Autodesk Fusion 360 part; units mm, degrees
(part 4 of 13)
  line L2684 (147.36, -101.854) -> (147.266, -101.874)
  line L2685 (145.516, -107.036) -> (145.448, -107.016)
  line L2686 (147.651, -101.836) -> (147.644, -101.834)
  line L2687 (148.011, -101.956) -> (148.011, -101.956)
  line L2688 (147.957, -106.91) -> (147.936, -106.978)
  line L2689 (147.447, -101.836) -> (147.36, -101.854)
  line L2690 (147.644, -101.834) -> (147.453, -101.834)
  line L2691 (147.999, -101.949) -> (147.999, -101.949)
  line L2692 (147.098, -101.949) -> (147.098, -101.949)
  line L2693 (147.651, -101.836) -> (147.651, -101.836)
  line L2694 (146.733, -102.004) -> (146.733, -102.004)
  line L2695 (146.733, -102.004) -> (146.727, -102.001)
  line L2696 (148.005, -101.952) -> (147.999, -101.949)
  line L2697 (146.727, -102.001) -> (146.633, -101.981)
  line L2698 (147.453, -101.834) -> (147.447, -101.836)
  line L2699 (146.342, -103.777) -> (146.349, -103.778)
  line L2700 (146.405, -103.778) -> (146.473, -103.799)
  line L2701 (146.349, -103.778) -> (146.405, -103.778)
  line L2702 (146.546, -101.963) -> (146.546, -101.963)
  line L2703 (147.936, -106.978) -> (147.883, -107.024)
  line L2704 (146.342, -101.963) -> (146.342, -101.963)
  line L2705 (145.448, -107.016) -> (145.402, -106.962)
  line L2706 (145.402, -106.962) -> (145.392, -106.892)
  line L2707 (146.255, -103.759) -> (146.342, -103.777)
  line L2708 (146.156, -103.736) -> (146.162, -103.739)
  line L2709 (145.844, -103.557) -> (145.988, -103.661)
  line L2710 (146.224, -101.988) -> (145.844, -102.369)
  line L2711 (146.54, -101.962) -> (146.349, -101.962)
  line L2712 (145.844, -102.369) -> (145.844, -103.557)
  line L2713 (146.473, -103.799) -> (146.494, -103.815)
  line L2714 (146.255, -101.981) -> (146.224, -101.988)
  line L2715 (146.546, -101.963) -> (146.54, -101.962)
  line L2716 (145.994, -103.664) -> (146.156, -103.736)
  line L2717 (146.342, -101.963) -> (146.255, -101.981)
  line L2718 (146.162, -103.739) -> (146.255, -103.759)
  line L2719 (146.342, -103.777) -> (146.342, -103.777)
  line L2720 (145.419, -106.809) -> (145.425, -106.765)
  line L2721 (146.173, -98.3593) -> (146.176, -98.3565)
  line L2722 (145.404, -106.846) -> (145.411, -106.828)
  line L2723 (145.994, -103.664) -> (145.994, -103.664)
  line L2724 (145.401, -106.858) -> (145.404, -106.846)
  line L2725 (145.415, -106.816) -> (145.419, -106.809)
  line L2726 (145.425, -106.765) -> (145.428, -106.754)
  line L2727 (145.398, -106.868) -> (145.399, -106.866)
  line L2728 (150.849, -79.1963) -> (150.82, -79.1551)
  line L2729 (150.946, -80.2588) -> (151.001, -80.0568)
  line L2730 (150.485, -80.0187) -> (150.435, -80.1497)
  line L2731 (150.946, -79.4056) -> (150.943, -79.3953)
  line L2732 (151.021, -79.8267) -> (151.002, -79.6184)
  line L2733 (150.821, -80.5085) -> (150.849, -80.4681)
  line L2734 (150.81, -79.1467) -> (150.796, -79.1537)
  line L2735 (151.002, -79.6184) -> (151.001, -79.6076)
  line L2736 (144.637, -93.3612) -> (144.728, -93.5556)
  line L2737 (144.879, -93.7872) -> (144.882, -93.7913)
  line L2738 (151.001, -79.6076) -> (150.946, -79.4056)
  line L2739 (144.568, -93.1202) -> (144.607, -93.2578)
  line L2740 (148.43, -96.7994) -> (148.43, -96.8204)
  line L2741 (148.43, -96.8204) -> (148.415, -96.8969)
  line L2742 (144.635, -93.3566) -> (144.637, -93.3612)
  line L2743 (144.607, -93.2578) -> (144.635, -93.3566)
  line L2744 (148.284, -97.5103) -> (148.289, -97.5255)
  line L2745 (144.637, -93.3612) -> (144.637, -93.3612)
  line L2746 (144.728, -93.5556) -> (144.741, -93.5839)
  line L2747 (144.744, -93.5881) -> (144.744, -93.5881)
  line L2748 (150.854, -80.4586) -> (150.943, -80.2691)
  line L2749 (150.797, -80.5114) -> (150.809, -80.5178)
  line L2750 (144.741, -93.5839) -> (144.744, -93.5881)
  line L2751 (145.25, -94.1228) -> (145.25, -94.1228)
  line L2752 (144.744, -93.5881) -> (144.879, -93.7872)
  line L2753 (150.796, -79.1537) -> (150.437, -79.5133)
  line L2754 (151.002, -80.046) -> (151.021, -79.8377)
  line L2755 (150.437, -79.5133) -> (150.49, -79.666)
  line L2756 (150.508, -79.8531) -> (150.485, -80.0187)
  line L2757 (150.809, -80.5178) -> (150.821, -80.5085)
  line L2758 (151.001, -80.0568) -> (151.002, -80.046)
  line L2759 (144.568, -93.1202) -> (144.568, -93.1202)
  line L2760 (146.166, -94.3699) -> (146.166, -94.3699)
  line L2761 (145.815, -94.3439) -> (145.955, -94.3681)
  line L2762 (146.346, -94.3555) -> (146.346, -94.3555)
  line L2763 (146.346, -94.3555) -> (146.351, -94.3551)
  line L2764 (145.988, -94.37) -> (145.988, -94.37)
  line L2765 (145.475, -94.2444) -> (145.48, -94.246)
  line L2766 (146.351, -94.3551) -> (146.356, -94.3539)
  line L2767 (150.943, -80.2691) -> (150.946, -80.2588)
  line L2768 (150.435, -80.1497) -> (150.797, -80.5114)
  line L2769 (150.943, -79.3953) -> (150.854, -79.2058)
  line L2770 (146.166, -94.3699) -> (146.346, -94.3555)
  line L2771 (145.329, -94.1662) -> (145.475, -94.2444)
  line L2772 (150.854, -79.2058) -> (150.849, -79.1963)
  line L2773 (144.882, -93.7913) -> (144.886, -93.795)
  line L2774 (145.712, -94.326) -> (145.815, -94.3439)
  line L2775 (151.021, -79.8377) -> (151.021, -79.8267)
  line L2776 (150.82, -79.1551) -> (150.81, -79.1467)
  line L2777 (150.849, -80.4681) -> (150.854, -80.4586)
  line L2778 (148.307, -97.0052) -> (148.284, -97.0097)
  line L2779 (144.879, -93.7872) -> (144.879, -93.7872)
  circle A28 centre (112.573, -110.134) radius 0.2
  circle A29 centre (123.749, -107.996) radius 0.2
  circle A30 centre (148.895, -97.028) radius 0.2
  circle A31 centre (115.214, -116.18) radius 0.2
  circle A32 centre (123.774, -112.954) radius 0.2
  circle A33 centre (92.8116, -81.2546) radius 0.2
  circle A34 centre (110.388, -108.255) radius 0.2
  circle A35 centre (131.47, -114.3) radius 0.2
  circle A36 centre (130.531, -107.975) radius 0.2
  circle A37 centre (137.897, -112.624) radius 0.2
  circle A38 centre (133.429, -109.717) radius 0.2
  circle A39 centre (150.622, -97.3582) radius 0.2
  circle A40 centre (128.067, -87.2236) radius 0.2
  circle A41 centre (146.228, -106.299) radius 0.2
  circle A42 centre (127.254, -107.061) radius 0.2
  circle A43 centre (115.113, -71.9328) radius 0.2
  circle A44 centre (105.74, -104.191) radius 0.2
  circle A45 centre (92.4814, -111.887) radius 0.2
  circle A46 centre (122.123, -94.5134) radius 0.2
  circle A47 centre (141.061, -112.152) radius 0.2
  circle A48 centre (92.4306, -104.216) radius 0.2
  circle A49 centre (115.214, -113.411) radius 0.2
  circle A50 centre (126.187, -110.49) radius 0.2
  circle A51 centre (126.749, -94.435) radius 0.2
  circle A52 centre (117.291, -131.755) radius 0.2
  circle A53 centre (136.169, -97.9424) radius 0.2
  circle A54 centre (138.735, -98.0186) radius 0.2
  circle A55 centre (132.232, -94.8763) radius 0.2
  circle A56 centre (147.701, -101.067) radius 0.2
  circle A57 centre (149.463, -102.253) radius 0.2
  circle A58 centre (144.958, -107.874) radius 0.2
  circle A59 centre (149.925, -95.573) radius 0.2
  circle A60 centre (123.901, -94.5134) radius 0.2
  circle A61 centre (147.549, -102.743) radius 0.2
  line L2780 (104.259, -121.194) -> (104.353, -121.345)
  circle A62 centre (126.543, -112.471) radius 0.2
  line L2781 (104.133, -121.067) -> (104.259, -121.194)
  line L2782 (104.132, -121.066) -> (104.133, -121.067)
  line L2783 (106.931, -109.689) -> (106.934, -109.709)
  line L2784 (106.805, -115.238) -> (104.132, -117.911)
  line L2785 (106.805, -109.476) -> (106.809, -109.48)
  line L2786 (106.809, -109.48) -> (106.839, -109.522)
  line L2787 (106.873, -109.56) -> (106.881, -109.579)
  line L2788 (106.951, -109.83) -> (106.951, -114.884)
  line L2789 (106.934, -109.709) -> (106.941, -109.728)
  line L2790 (106.951, -114.89) -> (106.944, -114.941)
  line L2791 (105.52, -108.191) -> (106.805, -109.476)
  line L2792 (106.869, -115.159) -> (106.836, -115.197)
  line L2793 (104.132, -117.911) -> (104.132, -121.066)
  line L2794 (106.951, -114.884) -> (106.951, -114.89)
  line L2795 (106.93, -115.03) -> (106.908, -115.077)
  line L2796 (106.881, -109.579) -> (106.893, -109.595)
  line L2797 (106.878, -115.14) -> (106.869, -115.159)
  line L2798 (106.94, -114.992) -> (106.933, -115.01)
  line L2799 (106.933, -115.01) -> (106.93, -115.03)
  line L2800 (106.941, -109.728) -> (106.944, -109.779)
  line L2801 (106.944, -114.941) -> (106.94, -114.992)
  line L2802 (103.077, -107.563) -> (103.096, -107.57)
  line L2803 (105.293, -108.064) -> (105.313, -108.067)
  line L2804 (107.04, -125.464) -> (107.072, -125.472)
  line L2805 (143.674, -125.474) -> (143.701, -125.474)
  line L2806 (106.992, -125.455) -> (106.992, -125.455)
  line L2807 (103.244, -107.634) -> (103.282, -107.667)
  line L2808 (105.441, -108.127) -> (105.479, -108.161)
  line L2809 (106.89, -115.124) -> (106.878, -115.14)
  line L2810 (106.893, -109.595) -> (106.91, -109.643)
  line L2811 (103.026, -107.559) -> (103.077, -107.563)
  line L2812 (143.609, -125.476) -> (143.609, -125.476)
  line L2813 (104.245, -122.205) -> (104.132, -122.312)
  line L2814 (143.583, -125.474) -> (143.594, -125.475)
  line L2815 (143.594, -125.475) -> (143.602, -125.477)
  line L2816 (106.944, -109.779) -> (106.951, -109.83)
  line L2817 (103.608, -107.982) -> (104.088, -107.982)
  line L2818 (105.223, -108.053) -> (105.274, -108.057)
  line L2819 (104.088, -107.982) -> (104.184, -108.001)
  line L2820 (107.072, -125.472) -> (107.083, -125.474)
  line L2821 (106.984, -125.454) -> (106.992, -125.455)
  line L2822 (106.992, -125.455) -> (107.028, -125.461)
  line L2823 (106.91, -109.643) -> (106.931, -109.689)
  line L2824 (104.132, -122.615) -> (106.962, -125.445)
  line L2825 (106.908, -115.077) -> (106.89, -115.124)
  line L2826 (103.116, -107.573) -> (103.162, -107.595)
  line L2827 (107.169, -125.477) -> (107.187, -125.475)
  line L2828 (103.21, -107.613) -> (103.226, -107.625)
  line L2829 (103.226, -107.625) -> (103.244, -107.634)
  line L2830 (104.353, -121.345) -> (104.412, -121.513)
  line L2831 (96.4732, -107.552) -> (96.4732, -107.502)
  line L2832 (107.198, -125.474) -> (143.583, -125.474)
  line L2833 (105.359, -108.088) -> (105.407, -108.106)
  line L2834 (104.184, -108.001) -> (104.249, -108.045)
  line L2835 (105.274, -108.057) -> (105.293, -108.064)
  line L2836 (105.167, -108.045) -> (105.173, -108.045)
  line L2837 (105.479, -108.161) -> (105.52, -108.191)
  line L2838 (104.249, -108.045) -> (105.167, -108.045)
  line L2839 (107.103, -125.474) -> (107.123, -125.476)
  line L2840 (104.407, -121.89) -> (104.344, -122.056)
  line L2841 (107.187, -125.475) -> (107.198, -125.474)
  line L2842 (103.162, -107.595) -> (103.21, -107.613)
  line L2843 (104.412, -121.513) -> (104.432, -121.691)
  line L2844 (105.313, -108.067) -> (105.359, -108.088)
  line L2845 (101.073, -107.552) -> (102.97, -107.552)
  line L2846 (105.173, -108.045) -> (105.223, -108.053)
  line L2847 (106.839, -109.522) -> (106.873, -109.56)
  line L2848 (107.15, -125.478) -> (107.169, -125.477)
  line L2849 (143.602, -125.477) -> (143.609, -125.476)
  line L2850 (103.282, -107.667) -> (103.323, -107.698)
  line L2851 (143.67, -125.475) -> (143.674, -125.474)
  line L2852 (94.3232, -107.552) -> (96.4732, -107.552)
  line L2853 (107.083, -125.474) -> (107.103, -125.474)
  line L2854 (103.096, -107.57) -> (103.116, -107.573)
  line L2855 (106.836, -115.197) -> (106.805, -115.238)
  line L2856 (107.143, -125.479) -> (107.15, -125.478)
  line L2857 (107.028, -125.461) -> (107.04, -125.464)
  line L2858 (102.976, -107.552) -> (103.026, -107.559)
  line L2859 (105.423, -108.118) -> (105.441, -108.127)
  line L2860 (143.609, -125.476) -> (143.67, -125.475)
  line L2861 (103.323, -107.698) -> (103.608, -107.982)
  line L2862 (101.073, -107.502) -> (101.073, -107.552)
  line L2863 (96.4732, -107.502) -> (101.073, -107.502)
  line L2864 (102.97, -107.552) -> (102.976, -107.552)
  line L2865 (105.407, -108.106) -> (105.423, -108.118)
  line L2866 (104.432, -121.713) -> (104.407, -121.89)
  line L2867 (147.946, -122.352) -> (147.95, -122.347)
  line L2868 (144.084, -125.317) -> (144.099, -125.306)
  line L2869 (147.652, -122.7) -> (147.656, -122.697)
  line L2870 (146.52, -122.967) -> (146.579, -122.983)
  line L2871 (143.8, -125.462) -> (143.813, -125.46)
  line L2872 (143.969, -125.401) -> (143.99, -125.386)
  line L2873 (147.83, -122.518) -> (147.946, -122.352)
  line L2874 (143.75, -125.472) -> (143.754, -125.472)
  line L2875 (147.464, -122.83) -> (147.469, -122.828)
  line L2876 (143.922, -125.423) -> (143.933, -125.417)
  line L2877 (147.261, -122.925) -> (147.304, -122.905)
  line L2878 (143.754, -125.472) -> (143.761, -125.472)
  line L2879 (147.952, -122.342) -> (147.952, -122.342)
  line L2880 (147.818, -122.535) -> (147.83, -122.518)
  line L2881 (143.873, -125.439) -> (143.908, -125.429)
  line L2882 (106.962, -125.445) -> (106.966, -125.446)
  line L2883 (143.761, -125.472) -> (143.781, -125.466)
  line L2884 (144.082, -125.318) -> (144.084, -125.317)
  line L2885 (144.015, -125.368) -> (144.046, -125.35)
  line L2886 (147.656, -122.697) -> (147.818, -122.535)
  line L2887 (146.579, -122.983) -> (146.584, -122.984)
  line L2888 (147.594, -122.741) -> (147.652, -122.7)
  line L2889 (143.781, -125.466) -> (143.8, -125.462)
  line L2890 (143.828, -125.457) -> (143.862, -125.443)
  line L2891 (146.584, -122.984) -> (146.812, -123.004)
  line L2892 (143.99, -125.386) -> (144.005, -125.375)
  line L2893 (143.705, -125.474) -> (143.705, -125.474)
  line L2894 (147.304, -122.905) -> (147.464, -122.83)
  line L2895 (143.908, -125.429) -> (143.908, -125.429)
  line L2896 (143.915, -125.427) -> (143.922, -125.423)
  line L2897 (104.132, -122.312) -> (104.132, -122.615)
  line L2898 (104.344, -122.056) -> (104.245, -122.205)
  line L2899 (147.952, -122.342) -> (148.044, -122.145)
  line L2900 (107.123, -125.476) -> (107.143, -125.479)
  line L2901 (143.828, -125.457) -> (143.828, -125.457)
  line L2902 (143.95, -125.408) -> (143.969, -125.401)
  line L2903 (146.812, -123.004) -> (147.04, -122.984)
  line L2904 (143.705, -125.474) -> (143.717, -125.473)
  line L2905 (144.046, -125.35) -> (144.053, -125.346)
  line L2906 (148.044, -122.145) -> (148.044, -122.145)
  line L2907 (147.04, -122.984) -> (147.045, -122.983)
  line L2908 (104.432, -121.691) -> (104.432, -121.713)
  line L2909 (144.053, -125.346) -> (144.067, -125.331)
  line L2910 (106.966, -125.446) -> (106.984, -125.454)
  line L2911 (143.813, -125.46) -> (143.813, -125.46)
  line L2912 (147.045, -122.983) -> (147.256, -122.926)
  line L2913 (143.933, -125.417) -> (143.95, -125.408)
  line L2914 (143.82, -125.459) -> (143.828, -125.457)
  line L2915 (144.067, -125.331) -> (144.082, -125.318)
  line L2916 (144.127, -125.272) -> (144.135, -125.264)
  line L2917 (147.652, -122.7) -> (147.652, -122.7)
  line L2918 (144.046, -125.35) -> (144.046, -125.35)
  line L2919 (143.862, -125.443) -> (143.873, -125.439)
  line L2920 (143.717, -125.473) -> (143.75, -125.472)
  line L2921 (146.399, -123) -> (146.461, -122.966)
  line L2922 (147.256, -122.926) -> (147.261, -122.925)
  line L2923 (143.908, -125.429) -> (143.915, -125.427)
  line L2924 (143.701, -125.474) -> (143.705, -125.474)
  line L2925 (143.922, -125.423) -> (143.922, -125.423)
  line L2926 (144.005, -125.375) -> (144.015, -125.368)
  line L2927 (143.813, -125.46) -> (143.82, -125.459)
  line L2928 (144.099, -125.306) -> (144.127, -125.272)
  line L2929 (144.135, -125.264) -> (146.399, -123)
  line L2930 (150.834, -138.766) -> (150.829, -138.766)
  line L2931 (151.926, -138.995) -> (151.705, -138.877)
  line L2932 (151.191, -138.751) -> (151.016, -138.751)
  line L2933 (150.67, -138.805) -> (150.586, -138.826)
  line L2934 (151.7, -138.875) -> (151.473, -138.797)
  line L2935 (147.95, -121.034) -> (147.837, -120.874)
  line L2936 (151.365, -138.777) -> (151.225, -138.753)
  line L2937 (151.93, -138.998) -> (151.93, -138.998)
  line L2938 (152.509, -139.452) -> (152.439, -139.463)
  line L2939 (152.562, -139.405) -> (152.509, -139.452)
  line L2940 (147.884, -120.689) -> (147.941, -120.675)
  line L2941 (147.952, -121.039) -> (147.95, -121.034)
  line L2942 (146.461, -122.966) -> (146.52, -122.967)
  line L2943 (152.351, -139.409) -> (152.301, -139.334)
  line L2944 (152.439, -139.463) -> (152.374, -139.434)
  line L2945 (148.106, -121.919) -> (148.125, -121.691)
  line L2946 (147.469, -122.828) -> (147.594, -122.741)
  line L2947 (147.952, -121.039) -> (147.952, -121.039)
  line L2948 (147.832, -120.738) -> (147.884, -120.689)
  line L2949 (148.125, -121.691) -> (148.106, -121.463)
  line L2950 (152.301, -139.334) -> (152.298, -139.33)
  line L2951 (150.581, -138.828) -> (150.581, -138.828)
  line L2952 (151.221, -138.752) -> (151.217, -138.752)
  line L2953 (152.298, -139.33) -> (152.197, -139.223)
  line L2954 (152.455, -124.205) -> (152.582, -139.337)
  line L2955 (151.473, -138.797) -> (151.468, -138.795)
  line L2956 (147.815, -120.806) -> (147.832, -120.738)
  line L2957 (152.197, -139.223) -> (152.129, -139.151)
  line L2958 (151.7, -138.875) -> (151.7, -138.875)
  line L2959 (148.044, -122.145) -> (148.046, -122.14)
  line L2960 (152.426, -120.8) -> (152.455, -124.205)
  line L2961 (151.225, -138.753) -> (151.221, -138.752)
  line L2962 (151.468, -138.795) -> (151.365, -138.777)
  line L2963 (150.834, -138.766) -> (150.834, -138.766)
  line L2964 (147.045, -122.983) -> (147.045, -122.983)
  line L2965 (147.95, -122.347) -> (147.952, -122.342)
  line L2966 (152.374, -139.434) -> (152.351, -139.409)
  line L2967 (150.581, -138.828) -> (150.46, -138.879)
  line L2968 (152.369, -120.695) -> (152.415, -120.749)
  line L2969 (152.071, -139.106) -> (151.93, -138.998)
  line L2970 (151.217, -138.752) -> (151.217, -138.752)
  line L2971 (147.256, -122.926) -> (147.256, -122.926)
  line L2972 (148.046, -121.241) -> (147.968, -121.073)
  line L2973 (147.941, -120.675) -> (152.3, -120.675)
  line L2974 (150.824, -138.767) -> (150.67, -138.805)
  line L2975 (150.586, -138.826) -> (150.581, -138.828)
  line L2976 (146.579, -122.983) -> (146.579, -122.983)
  line L2977 (147.968, -121.073) -> (147.952, -121.039)
  line L2978 (152.3, -120.675) -> (152.369, -120.695)
  line L2979 (152.415, -120.749) -> (152.426, -120.8)
  line L2980 (151.016, -138.751) -> (151.014, -138.751)
  line L2981 (148.106, -121.463) -> (148.046, -121.241)
  line L2982 (152.582, -139.337) -> (152.562, -139.405)
  line L2983 (148.046, -122.14) -> (148.106, -121.919)
  line L2984 (151.192, -138.751) -> (151.191, -138.751)
  line L2985 (150.829, -138.766) -> (150.824, -138.767)
  line L2986 (152.129, -139.151) -> (152.125, -139.148)
  line L2987 (152.125, -139.148) -> (152.071, -139.106)
  line L2988 (151.014, -138.751) -> (151.014, -138.751)
  line L2989 (147.837, -120.874) -> (147.815, -120.806)
  line L2990 (147.464, -122.83) -> (147.464, -122.83)
  line L2991 (151.705, -138.877) -> (151.7, -138.875)
  line L2992 (151.014, -138.751) -> (150.834, -138.766)
  line L2993 (149.864, -141.293) -> (149.964, -141.399)
  line L2994 (150.369, -141.781) -> (150.345, -141.848)
  line L2995 (149.616, -140.859) -> (149.616, -140.859)
  line L2996 (149.528, -140.114) -> (149.528, -140.119)
  line L2997 (97.264, -141.636) -> (97.2177, -141.582)
  line L2998 (150.037, -141.475) -> (150.037, -141.475)
  line L2999 (97.2131, -140.453) -> (97.2139, -140.314)
  line L3000 (150.037, -141.475) -> (150.228, -141.621)
  line L3001 (151.93, -138.998) -> (151.926, -138.995)
  line L3002 (150.033, -141.472) -> (150.037, -141.475)
  line L3003 (150.147, -139.055) -> (150.143, -139.058)
  line L3004 (149.545, -140.613) -> (149.547, -140.618)
  line L3005 (150.354, -141.712) -> (150.369, -141.781)
  line L3006 (149.517, -140.369) -> (149.517, -140.369)
  line L3007 (149.517, -140.369) -> (149.527, -140.45)
  line L3008 (149.616, -140.859) -> (149.675, -140.985)
  line L3009 (150.46, -138.879) -> (150.355, -138.924)
  line L3010 (149.524, -140.205) -> (149.517, -140.364)
  line L3011 (151.217, -138.752) -> (151.192, -138.751)
  line L3012 (150.228, -141.621) -> (150.228, -141.621)
  line L3013 (98.1577, -140.728) -> (98.1628, -140.729)
  line L3014 (150.228, -141.621) -> (150.232, -141.624)
  line L3015 (149.858, -141.285) -> (149.858, -141.285)
  line L3016 (97.5631, -140.38) -> (97.7413, -140.528)
  line L3017 (150.289, -141.891) -> (150.243, -141.899)
  line L3018 (150.351, -138.927) -> (150.147, -139.055)
  line L3019 (149.723, -141.086) -> (149.858, -141.285)
  line L3020 (150.355, -138.924) -> (150.351, -138.927)
  line L3021 (149.669, -139.634) -> (149.579, -139.868)
  line L3022 (149.545, -140.032) -> (149.528, -140.114)
  line L3023 (149.527, -140.45) -> (149.545, -140.613)
  line L3024 (98.1628, -140.729) -> (98.1628, -140.729)
  line L3025 (149.795, -139.417) -> (149.669, -139.634)
  line L3026 (149.528, -140.119) -> (149.524, -140.205)
  line L3027 (149.675, -140.985) -> (149.72, -141.082)
  line L3028 (149.723, -141.086) -> (149.723, -141.086)
  line L3029 (97.2883, -140.2) -> (97.3586, -140.191)
  line L3030 (149.858, -141.285) -> (149.861, -141.289)
  line L3031 (149.528, -140.119) -> (149.528, -140.119)
  line L3032 (97.4352, -140.233) -> (97.5631, -140.38)
  line L3033 (97.7413, -140.528) -> (97.9413, -140.645)
  line L3034 (150.232, -141.624) -> (150.293, -141.656)
  line L3035 (149.72, -141.082) -> (149.723, -141.086)
  line L3036 (149.578, -139.873) -> (149.578, -139.873)
  line L3037 (150.243, -141.899) -> (97.332, -141.656)
  line L3038 (98.1628, -140.729) -> (98.2158, -140.74)
  line L3039 (149.579, -139.868) -> (149.578, -139.873)
  line L3040 (97.2343, -140.246) -> (97.2883, -140.2)
  line L3041 (97.423, -140.22) -> (97.4352, -140.233)
  line L3042 (149.547, -140.618) -> (149.593, -140.782)
  line L3043 (149.578, -139.873) -> (149.545, -140.032)
  line L3044 (149.864, -141.293) -> (149.864, -141.293)
  line L3045 (149.547, -140.618) -> (149.547, -140.618)
  line L3046 (150.143, -139.058) -> (149.954, -139.223)
  line L3047 (97.332, -141.656) -> (97.264, -141.636)
  line L3048 (151.225, -138.753) -> (151.225, -138.753)
  line L3049 (150.824, -138.767) -> (150.824, -138.767)
  line L3050 (149.517, -140.364) -> (149.517, -140.369)
  line L3051 (149.861, -141.289) -> (149.864, -141.293)
  line L3052 (149.614, -140.855) -> (149.616, -140.859)
  line L3053 (151.192, -138.751) -> (151.192, -138.751)
  line L3054 (149.593, -140.782) -> (149.614, -140.855)
  line L3055 (149.954, -139.223) -> (149.795, -139.417)
  line L3056 (101.055, -140.779) -> (101.151, -140.782)
  line L3057 (101.811, -140.587) -> (101.811, -140.587)
  line L3058 (100.703, -140.729) -> (100.756, -140.74)
  line L3059 (97.2066, -141.53) -> (97.2131, -140.453)
  line L3060 (98.8458, -140.753) -> (98.8508, -140.752)
  line L3061 (97.9413, -140.645) -> (98.1577, -140.728)
  line L3062 (99.719, -140.16) -> (99.775, -140.117)
  line L3063 (97.3586, -140.191) -> (97.423, -140.22)
  line L3064 (99.775, -140.117) -> (99.8457, -140.11)
  line L3065 (98.8508, -140.752) -> (98.8508, -140.752)
  line L3066 (99.0627, -140.688) -> (99.0677, -140.686)
  line L3067 (102.171, -140.282) -> (102.259, -140.16)
  line L3068 (99.6283, -140.287) -> (99.6313, -140.282)
  line L3069 (98.8508, -140.752) -> (99.0627, -140.688)
  line L3070 (99.2757, -140.585) -> (99.4642, -140.45)
  line L3071 (101.608, -140.686) -> (101.613, -140.684)
  line L3072 (102.259, -140.16) -> (102.315, -140.117)
  line L3073 (100.703, -140.729) -> (100.703, -140.729)
  line L3074 (99.271, -140.587) -> (99.2711, -140.587)
  line L3075 (100.481, -140.645) -> (100.698, -140.728)
  line L3076 (99.0677, -140.686) -> (99.0726, -140.684)
  line L3077 (101.234, -140.772) -> (101.386, -140.753)
  line L3078 (102.315, -140.117) -> (102.386, -140.11)
  line L3079 (101.811, -140.587) -> (101.816, -140.585)
  line L3080 (98.3847, -140.774) -> (98.5153, -140.779)
  line L3081 (97.2177, -141.582) -> (97.2066, -141.53)
  line L3082 (98.6943, -140.772) -> (98.8458, -140.753)
  line L3083 (98.5153, -140.779) -> (98.6109, -140.782)
  line L3084 (100.756, -140.74) -> (100.925, -140.774)
  line L3085 (150.293, -141.656) -> (150.303, -141.662)
  line L3086 (98.6212, -140.782) -> (98.6212, -140.782)
  line L3087 (99.9488, -140.201) -> (99.9488, -140.201)
  line L3088 (97.2139, -140.314) -> (97.2343, -140.246)
  line L3089 (98.6212, -140.782) -> (98.6943, -140.772)
  line L3090 (98.2158, -140.74) -> (98.3847, -140.774)
  line L3091 (99.6313, -140.282) -> (99.719, -140.16)
  line L3092 (98.6109, -140.782) -> (98.611, -140.782)
  line L3093 (99.8457, -140.11) -> (99.9086, -140.143)
  line L3094 (102.469, -140.168) -> (102.489, -140.201)
  line L3095 (102.489, -140.201) -> (102.489, -140.201)
  line L3096 (100.698, -140.728) -> (100.703, -140.729)
  line L3097 (101.386, -140.753) -> (101.391, -140.752)
  line L3098 (102.386, -140.11) -> (102.449, -140.143)
  line L3099 (150.345, -141.848) -> (150.289, -141.891)
  line L3100 (99.9287, -140.168) -> (99.9488, -140.201)
  line L3101 (100.281, -140.528) -> (100.481, -140.645)
  line L3102 (101.161, -140.782) -> (101.234, -140.772)
  line L3103 (100.103, -140.38) -> (100.281, -140.528)
  line L3104 (99.2711, -140.587) -> (99.2757, -140.585)
  line L3105 (101.391, -140.752) -> (101.391, -140.752)
  line L3106 (101.816, -140.585) -> (102.004, -140.45)
  line L3107 (149.964, -141.399) -> (150.033, -141.472)
  line L3108 (99.9488, -140.201) -> (99.9515, -140.205)
  line L3109 (99.0726, -140.684) -> (99.271, -140.587)
  line L3110 (99.6313, -140.282) -> (99.6313, -140.282)
  line L3111 (99.9515, -140.205) -> (100.103, -140.38)
  line L3112 (99.9086, -140.143) -> (99.9287, -140.168)
  line L3113 (98.611, -140.782) -> (98.6161, -140.782)
  line L3114 (98.6161, -140.782) -> (98.6212, -140.782)
  line L3115 (150.303, -141.662) -> (150.354, -141.712)
  line L3116 (102.449, -140.143) -> (102.469, -140.168)
  line L3117 (99.4642, -140.45) -> (99.6283, -140.287)
  line L3118 (101.161, -140.782) -> (101.161, -140.782)
  line L3119 (101.156, -140.782) -> (101.161, -140.782)
  line L3120 (106.471, -140.752) -> (106.683, -140.688)
  line L3121 (102.171, -140.282) -> (102.171, -140.282)
  line L3122 (101.151, -140.782) -> (101.151, -140.782)
  line L3123 (103.691, -140.782) -> (103.696, -140.782)
  line L3124 (104.708, -140.287) -> (104.711, -140.282)
  line L3125 (102.168, -140.287) -> (102.171, -140.282)
  line L3126 (106.231, -140.782) -> (106.236, -140.782)
  line L3127 (106.314, -140.772) -> (106.466, -140.753)
  line L3128 (103.696, -140.782) -> (103.701, -140.782)
  line L3129 (105.361, -140.528) -> (105.561, -140.645)
  line L3130 (102.489, -140.201) -> (102.492, -140.205)
  line L3131 (106.693, -140.684) -> (106.891, -140.587)
  line L3132 (104.153, -140.684) -> (104.351, -140.587)
  line L3133 (105.029, -140.201) -> (105.029, -140.201)
  line L3134 (106.135, -140.779) -> (106.231, -140.782)
  line L3135 (103.243, -140.729) -> (103.243, -140.729)
  line L3136 (104.711, -140.282) -> (104.799, -140.16)
  line L3137 (104.926, -140.11) -> (104.989, -140.143)
  line L3138 (103.701, -140.782) -> (103.701, -140.782)
  line L3139 (105.783, -140.729) -> (105.836, -140.74)
  line L3140 (106.241, -140.782) -> (106.314, -140.772)
  line L3141 (105.778, -140.728) -> (105.783, -140.729)
  line L3142 (101.613, -140.684) -> (101.811, -140.587)
  line L3143 (105.183, -140.38) -> (105.361, -140.528)
  line L3144 (105.029, -140.201) -> (105.032, -140.205)
  line L3145 (103.701, -140.782) -> (103.774, -140.772)
  line L3146 (102.821, -140.528) -> (103.021, -140.645)
  line L3147 (100.925, -140.774) -> (101.055, -140.779)
  line L3148 (103.243, -140.729) -> (103.296, -140.74)
  line L3149 (101.151, -140.782) -> (101.156, -140.782)
  line L3150 (101.391, -140.752) -> (101.603, -140.688)
  line L3151 (103.595, -140.779) -> (103.691, -140.782)
  line L3152 (102.492, -140.205) -> (102.643, -140.38)
  line L3153 (103.931, -140.752) -> (104.143, -140.688)
  line L3154 (104.855, -140.117) -> (104.926, -140.11)
  line L3155 (101.603, -140.688) -> (101.608, -140.686)
  line L3156 (104.544, -140.45) -> (104.708, -140.287)
  line L3157 (104.799, -140.16) -> (104.855, -140.117)
  line L3158 (104.148, -140.686) -> (104.153, -140.684)
  line L3159 (103.774, -140.772) -> (103.926, -140.753)
  line L3160 (104.143, -140.688) -> (104.148, -140.686)
  line L3161 (103.926, -140.753) -> (103.931, -140.752)
  line L3162 (106.466, -140.753) -> (106.471, -140.752)
  line L3163 (104.351, -140.587) -> (104.351, -140.587)
  line L3164 (102.004, -140.45) -> (102.168, -140.287)
  line L3165 (105.783, -140.729) -> (105.783, -140.729)
  line L3166 (103.296, -140.74) -> (103.465, -140.774)
  line L3167 (102.643, -140.38) -> (102.821, -140.528)
  line L3168 (103.691, -140.782) -> (103.691, -140.782)
  line L3169 (104.989, -140.143) -> (105.009, -140.168)
  line L3170 (106.683, -140.688) -> (106.688, -140.686)
  line L3171 (104.356, -140.585) -> (104.544, -140.45)
  line L3172 (105.561, -140.645) -> (105.778, -140.728)
  line L3173 (106.891, -140.587) -> (106.896, -140.585)
  line L3174 (106.231, -140.782) -> (106.231, -140.782)
  line L3175 (106.471, -140.752) -> (106.471, -140.752)
  line L3176 (103.465, -140.774) -> (103.595, -140.779)
  line L3177 (103.931, -140.752) -> (103.931, -140.752)
  line L3178 (104.711, -140.282) -> (104.711, -140.282)
  line L3179 (106.688, -140.686) -> (106.693, -140.684)
  line L3180 (105.836, -140.74) -> (106.005, -140.774)
  line L3181 (104.351, -140.587) -> (104.356, -140.585)
  line L3182 (103.021, -140.645) -> (103.238, -140.728)
  line L3183 (103.238, -140.728) -> (103.243, -140.729)
  line L3184 (110.109, -140.201) -> (110.109, -140.201)
  line L3185 (110.641, -140.645) -> (110.858, -140.728)
  line L3186 (111.551, -140.752) -> (111.763, -140.688)
  line L3187 (107.339, -140.16) -> (107.395, -140.117)
  line L3188 (109.011, -140.752) -> (109.011, -140.752)
  line L3189 (109.223, -140.688) -> (109.228, -140.686)
  line L3190 (108.854, -140.772) -> (109.006, -140.753)
  line L3191 (108.781, -140.782) -> (108.854, -140.772)
  line L3192 (109.233, -140.684) -> (109.431, -140.587)
  line L3193 (106.005, -140.774) -> (106.135, -140.779)
  line L3194 (108.771, -140.782) -> (108.776, -140.782)
  line L3195 (108.323, -140.729) -> (108.323, -140.729)
  line L3196 (109.011, -140.752) -> (109.223, -140.688)
  line L3197 (107.251, -140.282) -> (107.251, -140.282)
  line L3198 (110.112, -140.205) -> (110.263, -140.38)
  line L3199 (107.901, -140.528) -> (108.101, -140.645)
  line L3200 (110.863, -140.729) -> (110.916, -140.74)
  line L3201 (111.311, -140.782) -> (111.316, -140.782)
  line L3202 (111.551, -140.752) -> (111.551, -140.752)
  line L3203 (106.236, -140.782) -> (106.241, -140.782)
  line L3204 (107.084, -140.45) -> (107.248, -140.287)
  line L3205 (106.891, -140.587) -> (106.891, -140.587)
  line L3206 (108.545, -140.774) -> (108.675, -140.779)
  line L3207 (108.318, -140.728) -> (108.323, -140.729)
  line L3208 (107.466, -140.11) -> (107.529, -140.143)
  line L3209 (107.395, -140.117) -> (107.466, -140.11)
  line L3210 (108.101, -140.645) -> (108.318, -140.728)
  line L3211 (111.546, -140.753) -> (111.551, -140.752)
  line L3212 (107.248, -140.287) -> (107.251, -140.282)
  line L3213 (105.009, -140.168) -> (105.029, -140.201)
  line L3214 (107.251, -140.282) -> (107.339, -140.16)
  line L3215 (109.431, -140.587) -> (109.431, -140.587)
  line L3216 (106.241, -140.782) -> (106.241, -140.782)
  line L3217 (107.572, -140.205) -> (107.723, -140.38)
  line L3218 (109.228, -140.686) -> (109.233, -140.684)
  line L3219 (110.069, -140.143) -> (110.089, -140.168)
  line L3220 (110.089, -140.168) -> (110.109, -140.201)
  line L3221 (110.109, -140.201) -> (110.112, -140.205)
  line L3222 (108.781, -140.782) -> (108.781, -140.782)
  line L3223 (108.776, -140.782) -> (108.781, -140.782)
  line L3224 (111.321, -140.782) -> (111.321, -140.782)
  line L3225 (109.791, -140.282) -> (109.879, -140.16)
  line L3226 (108.376, -140.74) -> (108.545, -140.774)
  line L3227 (107.723, -140.38) -> (107.901, -140.528)
  line L3228 (110.441, -140.528) -> (110.641, -140.645)
  line L3229 (108.771, -140.782) -> (108.771, -140.782)
  line L3230 (109.006, -140.753) -> (109.011, -140.752)
  line L3231 (106.896, -140.585) -> (107.084, -140.45)
  line L3232 (107.529, -140.143) -> (107.549, -140.168)
  line L3233 (107.569, -140.201) -> (107.572, -140.205)
  line L3234 (108.323, -140.729) -> (108.376, -140.74)
  line L3235 (105.032, -140.205) -> (105.183, -140.38)
  line L3236 (107.549, -140.168) -> (107.569, -140.201)
  line L3237 (108.675, -140.779) -> (108.771, -140.782)
  line L3238 (109.791, -140.282) -> (109.791, -140.282)
  line L3239 (107.569, -140.201) -> (107.569, -140.201)
  line L3240 (109.879, -140.16) -> (109.935, -140.117)
  line L3241 (110.858, -140.728) -> (110.863, -140.729)
  line L3242 (115.68, -140.51) -> (115.68, -140.51)
  line L3243 (109.624, -140.45) -> (109.788, -140.287)
  line L3244 (113.934, -140.772) -> (114.086, -140.753)
  line L3245 (114.313, -140.684) -> (114.511, -140.587)
  line L3246 (114.704, -140.45) -> (114.868, -140.287)
  line L3247 (111.321, -140.782) -> (111.394, -140.772)
  line L3248 (112.328, -140.287) -> (112.331, -140.282)
  line L3249 (112.546, -140.11) -> (112.609, -140.143)
  line L3250 (111.763, -140.688) -> (111.768, -140.686)
  line L3251 (112.649, -140.201) -> (112.652, -140.205)
  line L3252 (109.431, -140.587) -> (109.436, -140.585)
  line L3253 (111.971, -140.587) -> (111.971, -140.587)
  line L3254 (114.511, -140.587) -> (114.516, -140.585)
  line L3255 (115.888, -140.606) -> (115.888, -140.606)
  line L3256 (111.773, -140.684) -> (111.971, -140.587)
  line L3257 (115.888, -140.606) -> (116.099, -140.663)
  line L3258 (111.316, -140.782) -> (111.321, -140.782)
  line L3259 (111.215, -140.779) -> (111.311, -140.782)
  line L3260 (111.394, -140.772) -> (111.546, -140.753)
  line L3261 (112.475, -140.117) -> (112.546, -140.11)
  line L3262 (110.916, -140.74) -> (111.085, -140.774)
  line L3263 (109.788, -140.287) -> (109.791, -140.282)
  line L3264 (111.768, -140.686) -> (111.773, -140.684)
  line L3265 (113.625, -140.774) -> (113.755, -140.779)
  line L3266 (113.755, -140.779) -> (113.851, -140.782)
  line L3267 (113.861, -140.782) -> (113.934, -140.772)
  line L3268 (112.629, -140.168) -> (112.649, -140.201)
  line L3269 (112.331, -140.282) -> (112.419, -140.16)
  line L3270 (114.516, -140.585) -> (114.704, -140.45)
  line L3271 (110.263, -140.38) -> (110.441, -140.528)
  line L3272 (113.181, -140.645) -> (113.398, -140.728)
  line L3273 (112.419, -140.16) -> (112.475, -140.117)
  line L3274 (113.851, -140.782) -> (113.856, -140.782)
  line L3275 (114.091, -140.752) -> (114.303, -140.688)
  line L3276 (113.856, -140.782) -> (113.861, -140.782)
  line L3277 (112.649, -140.201) -> (112.649, -140.201)
  line L3278 (113.861, -140.782) -> (113.861, -140.782)
  line L3279 (114.868, -140.287) -> (115.003, -140.099)
  line L3280 (112.652, -140.205) -> (112.803, -140.38)
  line L3281 (112.803, -140.38) -> (112.981, -140.528)
  line L3282 (115.057, -140.035) -> (115.126, -140.017)
  line L3283 (115.193, -140.039) -> (115.225, -140.071)
  line L3284 (116.099, -140.663) -> (116.099, -140.663)
  line L3285 (111.971, -140.587) -> (111.976, -140.585)
  line L3286 (115.309, -140.191) -> (115.326, -140.215)
  line L3287 (113.398, -140.728) -> (113.403, -140.729)
  line L3288 (110.006, -140.11) -> (110.069, -140.143)
  line L3289 (111.085, -140.774) -> (111.215, -140.779)
  line L3290 (109.436, -140.585) -> (109.624, -140.45)
  line L3291 (110.863, -140.729) -> (110.863, -140.729)
  line L3292 (112.609, -140.143) -> (112.629, -140.168)
  line L3293 (115.493, -140.38) -> (115.675, -140.508)
  line L3294 (112.331, -140.282) -> (112.331, -140.282)
  line L3295 (113.403, -140.729) -> (113.403, -140.729)
  line L3296 (109.935, -140.117) -> (110.006, -140.11)
  line L3297 (113.851, -140.782) -> (113.851, -140.782)
  line L3298 (113.456, -140.74) -> (113.625, -140.774)
  line L3299 (111.311, -140.782) -> (111.311, -140.782)
  line L3300 (112.981, -140.528) -> (113.181, -140.645)
  line L3301 (112.164, -140.45) -> (112.328, -140.287)
  line L3302 (111.976, -140.585) -> (112.164, -140.45)
  line L3303 (114.086, -140.753) -> (114.091, -140.752)
  line L3304 (113.403, -140.729) -> (113.456, -140.74)
  line L3305 (115.003, -140.099) -> (115.009, -140.087)
  line L3306 (118.379, -140.585) -> (118.423, -140.605)
  line L3307 (117.732, -140.022) -> (117.734, -140.027)
  line L3308 (117.171, -140.38) -> (117.172, -140.38)
  line L3309 (119.524, -140.51) -> (119.524, -140.51)
  line L3310 (118.644, -140.664) -> (118.872, -140.684)
  line L3311 (116.104, -140.664) -> (116.332, -140.684)
  line L3312 (119.716, -140.377) -> (119.878, -140.215)
  line L3313 (119.529, -140.508) -> (119.711, -140.38)
  line L3314 (115.488, -140.377) -> (115.492, -140.38)
  line L3315 (114.303, -140.688) -> (114.308, -140.686)
  line L3316 (115.675, -140.508) -> (115.68, -140.51)
  line L3317 (115.839, -140.585) -> (115.883, -140.605)
  line L3318 (118.028, -140.377) -> (118.032, -140.38)
  line L3319 (116.776, -140.606) -> (116.776, -140.606)
  line L3320 (117.176, -140.377) -> (117.338, -140.215)
  line L3321 (115.326, -140.215) -> (115.488, -140.377)
  line L3322 (114.308, -140.686) -> (114.313, -140.684)
  line L3323 (117.734, -140.027) -> (117.866, -140.215)
  line L3324 (117.535, -139.935) -> (117.603, -139.915)
  line L3325 (120.028, -139.988) -> (120.075, -139.935)
  line L3326 (118.215, -140.508) -> (118.22, -140.51)
  line L3327 (118.033, -140.38) -> (118.215, -140.508)
  line L3328 (116.984, -140.51) -> (116.989, -140.508)
  line L3329 (117.732, -140.022) -> (117.732, -140.022)
  line L3330 (119.365, -140.585) -> (119.524, -140.51)
  line L3331 (117.472, -140.022) -> (117.488, -139.988)
  line L3332 (119.878, -140.215) -> (120.01, -140.027)
  line L3333 (115.225, -140.071) -> (115.309, -140.191)
  line L3334 (116.781, -140.605) -> (116.825, -140.585)
  line L3335 (115.492, -140.38) -> (115.492, -140.38)
  line L3336 (116.56, -140.664) -> (116.565, -140.663)
  line L3337 (116.776, -140.606) -> (116.781, -140.605)
  line L3338 (117.172, -140.38) -> (117.176, -140.377)
  line L3339 (117.866, -140.215) -> (118.028, -140.377)
  line L3340 (115.492, -140.38) -> (115.493, -140.38)
  line L3341 (117.472, -140.022) -> (117.472, -140.022)
  line L3342 (116.989, -140.508) -> (117.171, -140.38)
  line L3343 (115.009, -140.087) -> (115.057, -140.035)
  line L3344 (114.511, -140.587) -> (114.511, -140.587)
  line L3345 (116.332, -140.684) -> (116.56, -140.664)
  line L3346 (117.716, -139.988) -> (117.732, -140.022)
  line L3347 (116.984, -140.51) -> (116.984, -140.51)
  line L3348 (116.099, -140.663) -> (116.104, -140.664)
  line L3349 (117.172, -140.38) -> (117.172, -140.38)
  line L3350 (117.338, -140.215) -> (117.47, -140.027)
  line L3351 (120.01, -140.027) -> (120.012, -140.022)
  line L3352 (117.488, -139.988) -> (117.535, -139.935)
  line L3353 (116.825, -140.585) -> (116.984, -140.51)
  line L3354 (114.091, -140.752) -> (114.091, -140.752)
  line L3355 (115.68, -140.51) -> (115.839, -140.585)
  line L3356 (117.47, -140.027) -> (117.472, -140.022)
  line L3357 (119.712, -140.38) -> (119.716, -140.377)
  line L3358 (118.639, -140.663) -> (118.639, -140.663)
  line L3359 (119.321, -140.605) -> (119.365, -140.585)
  line L3360 (118.22, -140.51) -> (118.379, -140.585)
  line L3361 (118.032, -140.38) -> (118.033, -140.38)
  line L3362 (115.883, -140.605) -> (115.888, -140.606)
  line L3363 (115.126, -140.017) -> (115.193, -140.039)
  line L3364 (116.565, -140.663) -> (116.776, -140.606)
  line L3365 (117.603, -139.915) -> (117.671, -139.936)
  line L3366 (119.316, -140.606) -> (119.316, -140.606)
  line L3367 (117.671, -139.936) -> (117.716, -139.988)
  line L3368 (116.565, -140.663) -> (116.565, -140.663)
  line L3369 (118.032, -140.38) -> (118.032, -140.38)
  line L3370 (122.615, -139.935) -> (122.683, -139.915)
  line L3371 (119.105, -140.663) -> (119.105, -140.663)
  line L3372 (121.412, -140.684) -> (121.64, -140.664)
  line L3373 (122.55, -140.027) -> (122.552, -140.022)
  line L3374 (123.108, -140.377) -> (123.112, -140.38)
  line L3375 (118.872, -140.684) -> (119.1, -140.664)
  line L3376 (123.459, -140.585) -> (123.503, -140.605)
  line L3377 (123.719, -140.663) -> (123.719, -140.663)
  line L3378 (118.639, -140.663) -> (118.644, -140.664)
  line L3379 (119.1, -140.664) -> (119.105, -140.663)
  line L3380 (119.711, -140.38) -> (119.712, -140.38)
  line L3381 (120.012, -140.022) -> (120.012, -140.022)
  line L3382 (121.856, -140.606) -> (121.856, -140.606)
  line L3383 (120.755, -140.508) -> (120.76, -140.51)
  line L3384 (120.968, -140.606) -> (121.179, -140.663)
  line L3385 (121.905, -140.585) -> (122.064, -140.51)
  line L3386 (122.064, -140.51) -> (122.069, -140.508)
  line L3387 (123.719, -140.663) -> (123.724, -140.664)
  line L3388 (121.645, -140.663) -> (121.645, -140.663)
  line L3389 (122.568, -139.988) -> (122.615, -139.935)
  line L3390 (122.552, -140.022) -> (122.568, -139.988)
  line L3391 (123.724, -140.664) -> (123.952, -140.684)
  line L3392 (120.272, -140.022) -> (120.274, -140.027)
  line L3393 (118.428, -140.606) -> (118.428, -140.606)
  line L3394 (123.3, -140.51) -> (123.459, -140.585)
  line L3395 (120.919, -140.585) -> (120.963, -140.605)
  line L3396 (121.64, -140.664) -> (121.645, -140.663)
  line L3397 (119.316, -140.606) -> (119.321, -140.605)
  line L3398 (121.184, -140.664) -> (121.412, -140.684)
  line L3399 (118.428, -140.606) -> (118.639, -140.663)
  line L3400 (120.573, -140.38) -> (120.755, -140.508)
  line L3401 (120.568, -140.377) -> (120.572, -140.38)
  line L3402 (120.963, -140.605) -> (120.968, -140.606)
  line L3403 (120.143, -139.915) -> (120.211, -139.936)
  line L3404 (119.524, -140.51) -> (119.529, -140.508)
  line L3405 (119.712, -140.38) -> (119.712, -140.38)
  line L3406 (121.645, -140.663) -> (121.856, -140.606)
  line L3407 (119.105, -140.663) -> (119.316, -140.606)
  line L3408 (118.423, -140.605) -> (118.428, -140.606)
  line L3409 (120.211, -139.936) -> (120.256, -139.988)
  line L3410 (121.861, -140.605) -> (121.905, -140.585)
  line L3411 (120.572, -140.38) -> (120.573, -140.38)
  line L3412 (120.272, -140.022) -> (120.272, -140.022)
  line L3413 (121.179, -140.663) -> (121.179, -140.663)
  line L3414 (121.179, -140.663) -> (121.184, -140.664)
  line L3415 (120.274, -140.027) -> (120.406, -140.215)
  line L3416 (120.76, -140.51) -> (120.76, -140.51)
  line L3417 (120.075, -139.935) -> (120.143, -139.915)
  line L3418 (120.012, -140.022) -> (120.028, -139.988)
  line L3419 (120.406, -140.215) -> (120.568, -140.377)
  line L3420 (122.064, -140.51) -> (122.064, -140.51)
  line L3421 (123.503, -140.605) -> (123.508, -140.606)
  line L3422 (123.508, -140.606) -> (123.508, -140.606)
  line L3423 (123.3, -140.51) -> (123.3, -140.51)
  line L3424 (123.508, -140.606) -> (123.719, -140.663)
  line L3425 (122.946, -140.215) -> (123.108, -140.377)
  line L3426 (118.22, -140.51) -> (118.22, -140.51)
  line L3427 (120.968, -140.606) -> (120.968, -140.606)
  line L3428 (120.76, -140.51) -> (120.919, -140.585)
  line L3429 (122.683, -139.915) -> (122.751, -139.936)
  line L3430 (122.751, -139.936) -> (122.796, -139.988)
  line L3431 (121.856, -140.606) -> (121.861, -140.605)
  line L3432 (120.256, -139.988) -> (120.272, -140.022)
  line L3433 (120.572, -140.38) -> (120.572, -140.38)
  line L3434 (122.552, -140.022) -> (122.552, -140.022)
  line L3435 (123.295, -140.508) -> (123.3, -140.51)
  line L3436 (122.252, -140.38) -> (122.256, -140.377)
  line L3437 (122.814, -140.027) -> (122.946, -140.215)
  line L3438 (122.812, -140.022) -> (122.812, -140.022)
  line L3439 (123.112, -140.38) -> (123.113, -140.38)
  line L3440 (122.251, -140.38) -> (122.252, -140.38)
  line L3441 (123.113, -140.38) -> (123.295, -140.508)
  line L3442 (127.336, -140.377) -> (127.498, -140.215)
  line L3443 (124.604, -140.51) -> (124.609, -140.508)
  line L3444 (124.609, -140.508) -> (124.791, -140.38)
  line L3445 (126.492, -140.684) -> (126.72, -140.664)
  line L3446 (125.486, -140.215) -> (125.648, -140.377)
  line L3447 (125.648, -140.377) -> (125.652, -140.38)
  line L3448 (126.936, -140.606) -> (126.941, -140.605)
  line L3449 (126.259, -140.663) -> (126.264, -140.664)
  line L3450 (126.048, -140.606) -> (126.259, -140.663)
  line L3451 (127.763, -139.915) -> (127.831, -139.936)
  line L3452 (125.155, -139.935) -> (125.223, -139.915)
  line L3453 (125.835, -140.508) -> (125.84, -140.51)
  line L3454 (125.652, -140.38) -> (125.653, -140.38)
  line L3455 (124.791, -140.38) -> (124.792, -140.38)
  line L3456 (127.144, -140.51) -> (127.144, -140.51)
  line L3457 (125.999, -140.585) -> (126.043, -140.605)
  line L3458 (124.396, -140.606) -> (124.396, -140.606)
  line L3459 (122.069, -140.508) -> (122.251, -140.38)
  line L3460 (124.396, -140.606) -> (124.401, -140.605)
  line L3461 (125.352, -140.022) -> (125.352, -140.022)
  line L3462 (124.18, -140.664) -> (124.185, -140.663)
  line L3463 (124.604, -140.51) -> (124.604, -140.51)
  line L3464 (124.445, -140.585) -> (124.604, -140.51)
  line L3465 (124.401, -140.605) -> (124.445, -140.585)
  line L3466 (123.952, -140.684) -> (124.18, -140.664)
  line L3467 (125.09, -140.027) -> (125.092, -140.022)
  line L3468 (125.223, -139.915) -> (125.291, -139.936)
  line L3469 (125.092, -140.022) -> (125.092, -140.022)
  line L3470 (127.331, -140.38) -> (127.332, -140.38)
  line L3471 (124.185, -140.663) -> (124.396, -140.606)
  line L3472 (125.354, -140.027) -> (125.486, -140.215)
  line L3473 (125.352, -140.022) -> (125.354, -140.027)
  line L3474 (127.648, -139.988) -> (127.695, -139.935)
  line L3475 (122.812, -140.022) -> (122.814, -140.027)
  line L3476 (125.84, -140.51) -> (125.999, -140.585)
  line L3477 (126.941, -140.605) -> (126.985, -140.585)
  line L3478 (122.252, -140.38) -> (122.252, -140.38)
  line L3479 (123.112, -140.38) -> (123.112, -140.38)
  line L3480 (122.256, -140.377) -> (122.418, -140.215)
  line L3481 (125.291, -139.936) -> (125.336, -139.988)
  line L3482 (127.632, -140.022) -> (127.632, -140.022)
  line L3483 (126.043, -140.605) -> (126.048, -140.606)
  line L3484 (127.632, -140.022) -> (127.648, -139.988)
  line L3485 (125.336, -139.988) -> (125.352, -140.022)
  line L3486 (127.498, -140.215) -> (127.63, -140.027)
  line L3487 (124.792, -140.38) -> (124.796, -140.377)
  line L3488 (125.108, -139.988) -> (125.155, -139.935)
  line L3489 (124.796, -140.377) -> (124.958, -140.215)
  line L3490 (125.653, -140.38) -> (125.835, -140.508)
  line L3491 (124.958, -140.215) -> (125.09, -140.027)
  line L3492 (126.259, -140.663) -> (126.259, -140.663)
  line L3493 (126.936, -140.606) -> (126.936, -140.606)
  line L3494 (126.048, -140.606) -> (126.048, -140.606)
  line L3495 (125.652, -140.38) -> (125.652, -140.38)
  line L3496 (124.792, -140.38) -> (124.792, -140.38)
  line L3497 (127.63, -140.027) -> (127.632, -140.022)
  line L3498 (127.695, -139.935) -> (127.763, -139.915)
  line L3499 (122.796, -139.988) -> (122.812, -140.022)
  line L3500 (124.185, -140.663) -> (124.185, -140.663)
  line L3501 (126.985, -140.585) -> (127.144, -140.51)
  line L3502 (126.725, -140.663) -> (126.936, -140.606)
  line L3503 (125.84, -140.51) -> (125.84, -140.51)
  line L3504 (122.418, -140.215) -> (122.55, -140.027)
  line L3505 (125.092, -140.022) -> (125.108, -139.988)
  line L3506 (126.725, -140.663) -> (126.725, -140.663)
  line L3507 (127.892, -140.022) -> (127.892, -140.022)
  line L3508 (131.8, -140.664) -> (131.805, -140.663)
  line L3509 (130.92, -140.51) -> (131.079, -140.585)
  line L3510 (131.344, -140.664) -> (131.572, -140.684)
  line L3511 (127.332, -140.38) -> (127.332, -140.38)
  line L3512 (128.375, -140.508) -> (128.38, -140.51)
  line L3513 (130.432, -140.022) -> (130.434, -140.027)
  line L3514 (126.264, -140.664) -> (126.492, -140.684)
  line L3515 (129.481, -140.605) -> (129.525, -140.585)
  line L3516 (128.188, -140.377) -> (128.192, -140.38)
  line L3517 (127.831, -139.936) -> (127.876, -139.988)
  line L3518 (129.689, -140.508) -> (129.871, -140.38)
  line L3519 (128.38, -140.51) -> (128.38, -140.51)
  line L3520 (130.188, -139.988) -> (130.235, -139.935)
  line L3521 (128.38, -140.51) -> (128.539, -140.585)
  line L3522 (129.265, -140.663) -> (129.265, -140.663)
  line L3523 (129.032, -140.684) -> (129.26, -140.664)
  line L3524 (128.193, -140.38) -> (128.375, -140.508)
  line L3525 (128.799, -140.663) -> (128.799, -140.663)
  line L3526 (129.872, -140.38) -> (129.872, -140.38)
  line L3527 (131.128, -140.606) -> (131.128, -140.606)
  line L3528 (130.915, -140.508) -> (130.92, -140.51)
  line L3529 (130.92, -140.51) -> (130.92, -140.51)
  line L3530 (127.332, -140.38) -> (127.336, -140.377)
  line L3531 (129.876, -140.377) -> (130.038, -140.215)
  line L3532 (127.144, -140.51) -> (127.149, -140.508)
  line L3533 (130.566, -140.215) -> (130.728, -140.377)
  line L3534 (130.172, -140.022) -> (130.172, -140.022)
  line L3535 (130.432, -140.022) -> (130.432, -140.022)
  line L3536 (128.026, -140.215) -> (128.188, -140.377)
  line L3537 (128.583, -140.605) -> (128.588, -140.606)
  line L3538 (128.539, -140.585) -> (128.583, -140.605)
  line L3539 (129.265, -140.663) -> (129.476, -140.606)
  line L3540 (127.894, -140.027) -> (128.026, -140.215)
  line L3541 (129.476, -140.606) -> (129.481, -140.605)
  line L3542 (128.799, -140.663) -> (128.804, -140.664)
  line L3543 (127.876, -139.988) -> (127.892, -140.022)
  line L3544 (129.525, -140.585) -> (129.684, -140.51)
  line L3545 (126.72, -140.664) -> (126.725, -140.663)
  line L3546 (129.684, -140.51) -> (129.689, -140.508)
  line L3547 (129.476, -140.606) -> (129.476, -140.606)
  line L3548 (129.871, -140.38) -> (129.872, -140.38)
  line L3549 (128.192, -140.38) -> (128.193, -140.38)